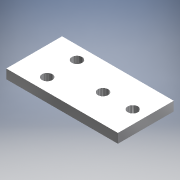
# Autodesk Inventor part: T-Bracing
Saved by Autodesk Inventor 2019.4 (Build 234330000, 330)
## iProperties
Created: 2020-01-03
Part Number: T-Bracing
Material: Aluminum 6061
Document SubType Name: Modeling
Designer: Mark
Mass: 23.0171 g
Surface Area: 46.5551 cm^2
Volume: 8.52483 cm^3
Density: 2.7 g/cm^3
Appearance: Aluminum - Flat
Author: Mark
Autodesk Inventor part; units mm, degrees
ref_plane "YZ Plane" through (0, 0, 0) normal (1, 0, 0) x (0, 1, 0)
ref_plane "XZ Plane" through (0, 0, 0) normal (0, 1, 0) x (-1, 0, 0)
ref_plane "XY Plane" through (0, 0, 0) normal (0, 0, 1) x (1, 0, 0)
sketch "Sketch1" plane through (0, 0, 0) normal (0, 1, 0) x (-1, 0, 0)
  line L0 (-15, 15) -> (15, 15)
  line L1 (15, 15) -> (15, -15)
  line L2 (15, -15) -> (-15, -15)
  line L3 (-15, -15) -> (-15, 15)
  line L4 (-15, 15) -> (15, -15) construction
  line L5 (15, 15) -> (-15, -15) construction
  circle A0 centre (0, 8) radius 2.75
  circle A1 centre (0, -8) radius 2.75
  line L6 (-45, 15) -> (-15, 15)
  line L7 (-15, 15) -> (-15, -15)
  line L8 (-15, -15) -> (-45, -15)
  line L9 (-45, -15) -> (-45, 15)
  line L10 (-45, 15) -> (-15, -15) construction
  line L11 (-15, 15) -> (-45, -15) construction
  circle A2 centre (-22, 0) radius 2.75
  circle A3 centre (-38, 0) radius 2.75
  point P0 (0, 0)
  point P1 (-30, 0)
  dimension "d0" = 30
  dimension "d1" = 30
  dimension "d2" = 5.5
  dimension "d3" = 5.5
  dimension "d4" = 15
  dimension "d5" = 15
  dimension "d6" = 7
  dimension "d7" = 7
  dimension "d8" = 30
  dimension "d9" = 30
  dimension "d10" = 5.5
  dimension "d11" = 5.5
  dimension "d12" = 15
  dimension "d13" = 15
  dimension "d14" = 7
  dimension "d15" = 7
  constraints: 24 end point, 4 centre point, 4 midpoint, 4 parallel, 2 collinear, 2 horizontal, 2 perpendicular
  measures "d0" distance of L1.end L2.end
  measures "d1" distance of L0.end L1.end
  measures "d2" diameter of A0
  measures "d3" diameter of A1
  measures "d4" distance from line of L1 A1.centre
  measures "d5" distance from line of L3 A0.centre
  measures "d6" distance from line of L0 A0.centre
  measures "d7" distance from line of L2 A1.centre
  measures "d8" distance of L7.end L8.end
  measures "d9" distance of L6.end L7.end
  measures "d10" diameter of A2
  measures "d11" diameter of A3
  measures "d12" distance from line of L8 A2.centre
  measures "d13" distance from line of L8 A3.centre
  measures "d14" distance from line of L3 A2.centre
  measures "d15" distance from line of L9 A3.centre
extrude "Extrusion1" add sketch "Sketch1" along normal blind 5
body "Solid1"
